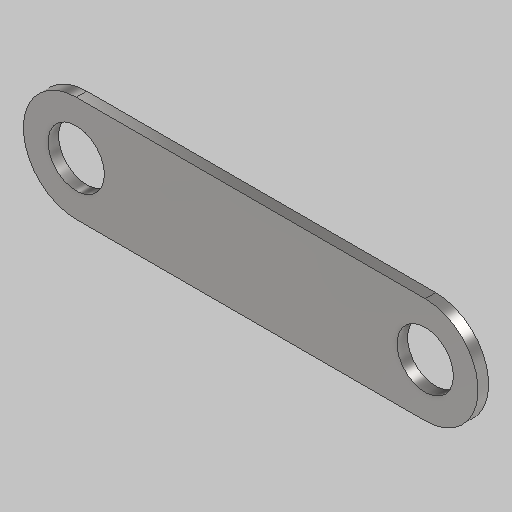
# Autodesk Inventor part: Chapa - Aperto fixação
Saved by Autodesk Inventor 2025.2 (Build 292293000, 293)
## iProperties
Created: 2024-05-02
Part Number: Chapa - Aperto fixação
Material: Genérico
Document SubType Name: Modeling
Designer: phmca
Density: 1 g/cm^3
Appearance: Padrão
Author: phmca
Autodesk Inventor part; units mm, degrees
ref_plane "YZ Plane" through (0, 0, 0) normal (1, 0, 0) x (0, 1, 0)
ref_plane "XZ Plane" through (0, 0, 0) normal (0, 1, 0) x (-1, 0, 0)
ref_plane "XY Plane" through (0, 0, 0) normal (0, 0, 1) x (1, 0, 0)
sketch "Esboço1" plane through (0, 0, 0) normal (0, 0, 1) x (1, 0, 0)
  line L0 (-49.5, 0) -> (49.5, 0) construction
  line L1 (-49.5, -15) -> (49.5, -15)
  line L2 (49.5, 15) -> (-49.5, 15)
  arc A0 (-49.5, 15) -> (-49.5, -15) centre (-49.5, 0) ccw
  arc A1 (49.5, -15) -> (49.5, 15) centre (49.5, 0) ccw
  circle A2 centre (-49.5, 0) radius 8
  circle A3 centre (49.5, 0) radius 8
  point P0 (0, 0)
  dimension "d0" = 16
  dimension "d1" = 99
  dimension "d4" = 30
  constraints: 8 end point, 4 centre point, 4 point on circle, 4 tangent, 2 coincident, 1 horizontal, 1 midpoint, 1 parallel
  measures "d0" diameter of A2
  measures "d1" distance of L0.end L0.start
  measures "d4" distance between parallel lines of L1 L2
extrude "Extrusão1" add sketch "Esboço1" along normal mid plane 3
sketch "Esboço2" plane through (0, 0, 1.5) normal (0, 0, 1) x (1, 0, 0)
  circle A0 centre (-49.5, 0) radius 8 projected
  circle A1 centre (49.5, 0) radius 8 projected
  line L0 (-49.5, 0) -> (49.5, 0)
  line L1 (0, 0) -> (0, -34.993)
  constraints: 4 end point, 1 horizontal, 1 vertical
